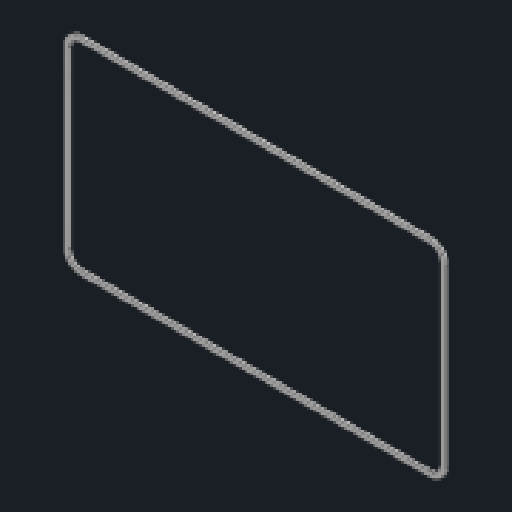
# Autodesk Inventor part: Rim
Saved by Autodesk Inventor 2024 (Build 280153000, 153)
## iProperties
Created: 2024-06-26
Part Number: Rim
Material: Generic
Document SubType Name: Modeling
Designer: Averey Ku
Density: 1 g/cm^3
Appearance: Default
Author: Averey Ku
Autodesk Inventor part; units mm, degrees
ref_plane "YZ Plane" through (0, 0, 0) normal (1, 0, 0) x (0, 1, 0)
ref_plane "XZ Plane" through (0, 0, 0) normal (0, 1, 0) x (-1, 0, 0)
ref_plane "XY Plane" through (0, 0, 0) normal (0, 0, 1) x (1, 0, 0)
sketch "Sketch1" plane through (0, 0, 0) normal (0, 0, 1) x (1, 0, 0)
  arc A0 (-57.15, -25.4) -> (-50.8, -31.75) centre (-50.8, -25.4) ccw projected
  line L0 (50.8, -31.75) -> (-50.8, -31.75) projected
  arc A1 (50.8, -31.75) -> (57.15, -25.4) centre (50.8, -25.4) ccw projected
  line L1 (57.15, 25.4) -> (57.15, -25.4) projected
  arc A2 (57.15, 25.4) -> (50.8, 31.75) centre (50.8, 25.4) ccw projected
  line L2 (-50.8, 31.75) -> (50.8, 31.75) projected
  arc A3 (-50.8, 31.75) -> (-57.15, 25.4) centre (-50.8, 25.4) ccw projected
  line L3 (-57.15, -25.4) -> (-57.15, 25.4) projected
  arc A4 (-50.8, 30.1625) -> (-55.5625, 25.4) centre (-50.8, 25.4) ccw
  line L4 (-50.8, 30.1625) -> (50.8, 30.1625)
  arc A5 (55.5625, 25.4) -> (50.8, 30.1625) centre (50.8, 25.4) ccw
  line L5 (55.5625, 25.4) -> (55.5625, -25.4)
  arc A6 (50.8, -30.1625) -> (55.5625, -25.4) centre (50.8, -25.4) ccw
  line L6 (50.8, -30.1625) -> (-50.8, -30.1625)
  arc A7 (-55.5625, -25.4) -> (-50.8, -30.1625) centre (-50.8, -25.4) ccw
  line L7 (-55.5625, -25.4) -> (-55.5625, 25.4)
  arc A8 (-50.8, 28.575) -> (-53.975, 25.4) centre (-50.8, 25.4) ccw
  line L8 (-50.8, 28.575) -> (50.8, 28.575)
  arc A9 (53.975, 25.4) -> (50.8, 28.575) centre (50.8, 25.4) ccw
  line L9 (53.975, 25.4) -> (53.975, -25.4)
  arc A10 (50.8, -28.575) -> (53.975, -25.4) centre (50.8, -25.4) ccw
  line L10 (50.8, -28.575) -> (-50.8, -28.575)
  arc A11 (-53.975, -25.4) -> (-50.8, -28.575) centre (-50.8, -25.4) ccw
  line L11 (-53.975, -25.4) -> (-53.975, 25.4)
  point P0 (0, 0)
  dimension "d0" = 1.5875
  constraints: 16 end point, 16 point on circle, 8 centre point, 14 other
  measures "d0" distance between parallel lines of L3 L7
extrude "Extrusion1" add sketch "Sketch1" along normal blind 0.762 contours L4 A5 L5 A6 L6 A7 L7 A4
body "Solid1"
